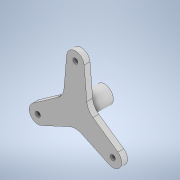
# Autodesk Inventor part: Shaft_output
Saved by Autodesk Inventor 2020 (Build 240168000, 168)
## iProperties
Created: 2020-05-11
Part Number: Shaft_output
Material: Generic
Document SubType Name: Modeling
Designer: avi41
Density: 1 g/cm^3
Appearance: Default
Author: avi41
Autodesk Inventor part; units mm, degrees
ref_plane "YZ Plane" through (0, 0, 0) normal (1, 0, 0) x (0, 1, 0)
ref_plane "XZ Plane" through (0, 0, 0) normal (0, 1, 0) x (-1, 0, 0)
ref_plane "XY Plane" through (0, 0, 0) normal (0, 0, 1) x (1, 0, 0)
sketch "Sketch1" plane through (0, 0, 0) normal (0, 1, 0) x (-1, 0, 0)
  line L0 (0, -27.5) -> (0, 7.5) construction
  line L1 (-54, 0) -> (9, 0) construction
  line L2 (0, 2.5) -> (-45, 2.5)
  line L3 (-45, 2.5) -> (-45, -2.5)
  line L4 (-45, -2.5) -> (-7.5, -2.5)
  line L5 (-7.5, -2.5) -> (-7.5, -22.5)
  line L6 (-7.5, -22.5) -> (0, -22.5)
  line L7 (0, -22.5) -> (0, 2.5)
  point P0 (0, 0)
  dimension "d0" = 7.5
  dimension "d1" = 5
  dimension "d4" = 45
  dimension "d5" = 20
  constraints: 12 end point, 4 perpendicular, 1 collinear, 1 horizontal, 1 point on line, 1 other
  measures "d0" distance of L5.end L6.end
  measures "d1" distance of L2.end L3.end
  measures "d4" distance between parallel lines of L0 L3
  measures "d5" distance between parallel lines of L4 L6
revolve "Revolution1" add sketch "Sketch1" angle 360 about axis through (0, 0, 0) along (0, 0, 1)
fillet "Fillet1" radius 2 1 edges at (-7.5, 0, -2.5)
sketch "Sketch2" plane through (0, 0, -2.5) normal (0, 0, -1) x (-1, 0, 0)
  line L0 (0, -63.2055) -> (0, 64.2333) construction
  line L1 (-63, 0) -> (63, 0) construction
  arc A0 (7.4715, 37.7287) -> (0, 44.575) centre (0, 37.075) ccw
  circle A1 centre (0, 0) radius 7.5 construction
  line L2 (0, 0) -> (38.9711, -22.5) construction
  circle A2 centre (0, 0) radius 45 projected
  line L3 (0, 0) -> (-38.9711, -22.5) construction
  line L4 (0, 0) -> (38.9711, 22.5)
  arc A3 (9.7463, 11.727) -> (11.3734, 6.5665) centre (22.1987, 12.8165) ccw
  line L5 (7.4715, 37.7287) -> (9.7463, 11.727)
  arc A4 (0, 44.575) -> (-7.4715, 37.7287) centre (0, 37.075) ccw
  arc A5 (-11.3734, 6.5665) -> (-9.7463, 11.727) centre (-22.1987, 12.8165) ccw
  line L6 (-7.4715, 37.7287) -> (-9.7463, 11.727)
  line L7 (0, 0) -> (-6.4952, 3.75)
  line L8 (-11.3734, 6.5665) -> (-38.9711, 22.5)
  circle A6 centre (0, 37.075) radius 2.1
  point P0 (-38.9711, 22.5)
  point P1 (0, 45)
  point P2 (0, 45)
  dimension "d6" = 15
  dimension "d7" = 120
  dimension "d8" = 120
  dimension "d9" = 60
  dimension "d10" = 60
  dimension "d11" = 37.075
  dimension "d12" = 25
  dimension "d13" = 5
  dimension "d19" = 4.2
  constraints: 14 end point, 11 point on circle, 5 centre point, 5 symmetric about line, 4 point on line, 2 tangent, 1 coincident, 4 other
  measures "d6" diameter of A0
  measures "d7" angle of L0 L3
  measures "d8" angle of L0 L2
  measures "d9" angle of L4 L0
  measures "d10" angle of L2 L4
  measures "d11" distance from line of L1 A0.centre
  measures "d12" diameter of A3
  measures "d13" angle of L5 L0
  measures "d19" diameter of A6
extrude "Extrusion1" cut sketch "Sketch2" against normal through all contours A0 A4 L6 A5 L8 A2 L4 A3 L5 | A6 picked at (-14.556, 28.6205)
pattern_circular "Circular Pattern1" count 3 over 360 about axis through (0, 0, -10) along (0, 0, 1) of "Extrusion1"
equation "\"d9\" = d10"
body "Solid1"
